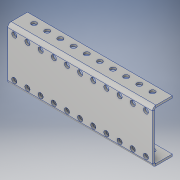
# Autodesk Inventor part: Intake back outer
Saved by Autodesk Inventor 2019 (Build 230136000, 136)
## iProperties
Created: 2018-11-07
Part Number: Intake back outer
Material: Aluminum 6061
Document SubType Name: Sheet Metal
Designer: woodk
Density: 2.7 g/cm^3
Sheet Metal Rule: Haakon
Appearance: Aluminum - Flat
Mass: 59.0331 g
Surface Area: 237.591 cm^2
Volume: 21.8641 cm^3
Author: woodk
Autodesk Inventor part; units mm, degrees
ref_plane "YZ Plane" through (0, 0, 0) normal (1, 0, 0) x (0, 1, 0)
ref_plane "XZ Plane" through (0, 0, 0) normal (0, 1, 0) x (-1, 0, 0)
ref_plane "XY Plane" through (0, 0, 0) normal (0, 0, 1) x (1, 0, 0)
sketch "Sketch1" plane through (0, 0, 0) normal (0, 0, 1) x (1, 0, 0)
  line L0 (0, 0) -> (139.7, 0)
  line L1 (139.7, 0) -> (139.7, 50.8)
  line L2 (139.7, 50.8) -> (0, 50.8)
  line L3 (0, 50.8) -> (0, 0)
  dimension "d0" = 50.8
  dimension "d1" = 139.7
  measures "d0" distance of L2.end L0.start
  measures "d1" distance of L0.start L0.end
extrude "Plate1" add sketch "Sketch1" along normal blind 2.032
sketch "Sketch2" plane through (139.7, 48.768, 2.032) normal (0, 1, 0) x (-1, 0, 0)
  line L0 (139.7, 0) -> (0, 0)
  line L1 (0, 0) -> (0, -19.05)
  line L2 (0, -19.05) -> (139.7, -19.05)
  line L3 (139.7, -19.05) -> (139.7, 0)
  constraints: 6 end point, 1 horizontal, 1 perpendicular, 1 vertical
edge flange "Flange1" height 19.05 angle 90 thickness 2.032 bend radius 1.27 thickness toward (0, 1, 0) relief tear relief width 2.032 relief depth 1.016 edges at (69.85, 50.8, 0) wall of the first edge with corners at (0, 48.768, 2.032) (139.7, 48.768, 2.032) (139.7, 48.768, -17.018) (0, 48.768, -17.018)
bend "Bend1"
corner "Corner1"
sketch "Sketch3" plane through (0, 2.032, 2.032) normal (0, -1, 0) x (1, 0, 0)
  line L0 (139.7, 0) -> (0, 0)
  line L1 (0, 0) -> (0, -19.05)
  line L2 (0, -19.05) -> (139.7, -19.05)
  line L3 (139.7, -19.05) -> (139.7, 0)
  constraints: 6 end point, 1 horizontal, 1 perpendicular, 1 vertical
edge flange "Flange2" height 19.05 angle 90 thickness 2.032 bend radius 1.27 thickness toward (0, -1, 0) relief tear relief width 2.032 relief depth 1.016 edges at (69.85, 0, 0) wall of the first edge with corners at (139.7, 2.032, 2.032) (0, 2.032, 2.032) (0, 2.032, -17.018) (139.7, 2.032, -17.018)
bend "Bend2"
corner "Corner2"
sketch "Sketch4" plane through (0, 0, 2.032) normal (0, 0, 1) x (1, 0, 0)
  line L0 (0, 3.302) -> (0, 47.498) projected
  line L1 (0, 50.8) -> (139.7, 50.8) projected
  line L2 (139.7, 0) -> (0, 0) projected
  point P0 (6.35, 44.45)
  point P1 (6.35, 6.35)
  dimension "d23" = 6.35
  dimension "d24" = 6.35
  dimension "d25" = 6.35
  constraints: 1 vertical alignment
  measures "d23" distance from line of L0 point (6.35, 44.45)
  measures "d24" distance from line of L1 point (6.35, 44.45)
  measures "d25" distance from line of L2 point (6.35, 6.35)
hole "Hole1" at (6.35, 44.45, 2.032) at (6.35, 6.35, 2.032) direction (0, 0, -1) diameter 4.9784 end through all
pattern_linear "Rectangular Pattern1" count 11 spacing 12.7 along (1, 0, 0) of "Hole1"
sketch "Sketch5" plane through (0, 50.8, -17.018) normal (0, 1, 0) x (1, 0, 0)
  line L0 (139.7, -19.05) -> (0, -19.05) projected
  line L1 (0, -15.748) -> (0, 0) projected
  point P0 (0, -17.018)
  point P1 (12.7, -6.35)
  dimension "d36" = 12.7
  dimension "d37" = 12.7
  measures "d36" distance from line of L0 point (12.7, -6.35)
  measures "d37" distance from line of L1 point (12.7, -6.35)
hole "Hole2" at (12.7, 50.8, -10.668) direction (0, -1, 0) diameter 4.9784 end through all
pattern_linear "Rectangular Pattern2" count 10 spacing 12.7 along (1, 0, 0) of "Hole2"
equation "\"d31\" = Thickness"
equation "\"d43\" = Thickness"
equation "\"d2\" = Thickness"
equation "\"d3\" = BendReliefWidth"
equation "\"d4\" = BendReliefDepth"
equation "\"d5\" = MinimumRemnant"
equation "\"d6\" = TransitionRadius"
equation "\"d9\" = BendRadius"
equation "\"d10\" = CornerReliefSize"
equation "\"d11\" = GapSize"
equation "\"d12\" = JacobiRadiusSize"
equation "\"d13\" = BendReliefWidth"
equation "\"d14\" = BendReliefDepth"
equation "\"d15\" = MinimumRemnant"
equation "\"d16\" = TransitionRadius"
equation "\"d19\" = BendRadius"
equation "\"d20\" = CornerReliefSize"
equation "\"d21\" = GapSize"
equation "\"d22\" = JacobiRadiusSize"
equation "\"BendReliefWidth\" = Thickness"
equation "\"BendReliefDepth\" = 0.5 * Thickness"
equation "\"CornerReliefSize\" = 4 * Thickness"
equation "\"MinimumRemnant\" = 2 * Thickness"
equation "\"TransitionRadius\" = BendRadius"
equation "\"JacobiRadiusSize\" = BendRadius"
equation "\"GapSize\" = Thickness"
equation "\"Thickness\" = 2.032"
equation "\"BendRadius\" = 1.27"
body "Solid1"
